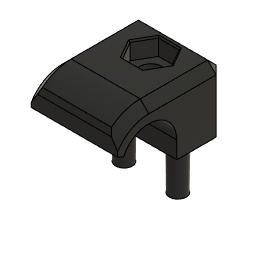
16mm Claw [(P)MPLA000000141] v1 (Autodesk Fusion 360 design; units mm, degrees)
Autodesk Fusion 360 part; units mm, degrees
sketch "Sketch1" plane through (0, 0, 0) normal (1, 0, 0) x (0, 1, 0)
  line L0 (7.7961, -6) -> (22, -6)
  line L1 (8.1, 0) -> (8.1, -8)
  circle A0 centre (0, 0) radius 11.1
  line L2 (0, 11.1) -> (22, 11.1)
  line L3 (22, 11.1) -> (22, -8)
  circle A1 centre (0, 0) radius 8.1
  line L4 (0, 0) -> (-8.1139, 8.1139)
  line L5 (0, 0) -> (-10.06, 4.6911)
  circle A2 centre (0, 0) radius 6.5
  circle A3 centre (0, 0) radius 13.1
  line L6 (-10.06, 4.6911) -> (-10.06, 9.7741)
  line L7 (0, 13.1) -> (22, 13.1)
  line L8 (22, 13.1) -> (22, 11.1)
  line L9 (-9.06, 4.2248) -> (-9.06, 9.7741)
  dimension "d179" = 3
  dimension "d181" = 16.2
  dimension "d182" = 20
  dimension "d6" = 5
  dimension "d33" = 22
  constraint concentric A1 A2
  constraint coincident A0.centre A1.centre
  constraint coincident L2.start A0
  constraint tangent A0 L2
  constraint vertical L3
  constraint coincident L5.end A0
  constraint coincident L0.end L3
  constraint perpendicular L0 L3
  constraint coincident L1.start A1
  constraint tangent L1 A1
  constraint vertical L6
  constraint coincident A3 L7.start
  constraint tangent A3 L7
  constraint perpendicular L3 L7
  constraint perpendicular L2 L8
  constraint parallel L6 L9
  constraint coincident L5 L9.start
  measures "d181" diameter of A1
  measures "d182" angle of L4 L5
  measures "d33" distance of A0.centre L3
extrude "Extrude1" add sketch "Sketch1" along normal mid plane 25 contours L0 L1 A0 A1 L4 | L0 A0 L2 A3 | L0 L2 L3 A3 | A0 A1 L4 L5 L9 | A0 L2 A3 L9 | L2 A3 L7 L8
sketch "Sketch2" plane through (0, 0, -6) normal (0, 0, -1) x (1, 0, 0)
  line L0 (-12.5, -22) -> (12.5, -22)
  line L1 (12.5, -22) -> (12.5, -8.1)
  line L2 (12.5, -8.1) -> (-12.5, -8.1)
  line L3 (-12.5, -8.1) -> (-12.5, -22)
  circle A0 centre (-11.3, 12.8) radius 2.55
  circle A1 centre (-11.3, 12.8) radius 1
  circle A2 centre (4.3, 12.8) radius 2.55
  circle A3 centre (4.3, 12.8) radius 1
  circle A4 centre (0, -13.1) radius 3.2
  circle A5 centre (-7.8, -13.1) radius 2.55
  circle A6 centre (-7.8, -13.1) radius 2.2
  circle A7 centre (7.8, -13.1) radius 2.55
  circle A8 centre (7.8, -13.1) radius 2.2
  dimension "d233" = 2
  dimension "d234" = 2
  dimension "d240" = 15.6
  dimension "d242" = 5.1
  dimension "d243" = 5.1
  dimension "d162" = 6.4
  dimension "d223" = 5.1
  dimension "d224" = 5.1
  dimension "d225" = 4.4
  dimension "d226" = 4.4
  dimension "d227" = 15.6
  dimension "d20" = 7.8
  dimension "d32" = 5
  constraint horizontal A0.centre A2.centre
  constraint concentric A2 A3
  constraint concentric A0 A1
  constraint concentric A7 A8
  constraint concentric A5 A6
  constraint horizontal A7.centre A4.centre
  constraint horizontal A5.centre A4.centre
  constraint vertical origin A4.centre
  measures "d233" diameter of A1
  measures "d234" diameter of A3
  measures "d240" distance of A0.centre A2.centre
  measures "d242" diameter of A2
  measures "d243" diameter of A0
  measures "d162" diameter of A4
  measures "d223" diameter of A7
  measures "d224" diameter of A5
  measures "d225" diameter of A8
  measures "d226" diameter of A6
  measures "d227" distance of A5.centre A7.centre
  measures "d20" distance of A7.centre A4.centre
  measures "d32" distance of L2 A7.centre
extrude "Extrude2" add sketch "Sketch2" along normal blind 12 contours A5 | A6 | A7 | A8
draft "Draft1" angle 0.5 neutral plane through (0, 11.6452, -6) pull (0, 0, -1) 2 faces at (-5.2532, 13.2271, -14) (10.3468, 13.2271, -14)
sketch "Sketch3" plane through (0, 0, -6) normal (0, 0, -1) x (1, 0, 0)
extrude "Extrude3" cut sketch "Sketch2" against normal blind 20 contours A4
sketch "Sketch4" plane through (0, 0, 13.1) normal (0, 0, 1) x (-1, 0, 0)
  circle A0 centre (0, -13.1) radius 3.2
  line L0 (12.5, 0) -> (-12.5, 0)
  line L1 (-12.5, 0) -> (-12.5, -22)
  line L2 (-12.5, -22) -> (12.5, -22)
  line L3 (12.5, -22) -> (12.5, 0)
  line L4 (3.0022, -18.3) -> (6.0044, -13.1)
  line L5 (6.0044, -13.1) -> (3.0022, -7.9)
  line L6 (3.0022, -7.9) -> (-3.0022, -7.9)
  line L7 (-3.0022, -7.9) -> (-6.0044, -13.1)
  line L8 (-6.0044, -13.1) -> (-3.0022, -18.3)
  line L9 (-3.0022, -18.3) -> (3.0022, -18.3)
  point P0 (0, -13.1)
  dimension "d27" = 5.2
  constraint coincident P0 A0.centre
  measures "d27" distance of P0 L9
extrude "Extrude4" cut sketch "Sketch4" against normal blind 5 contours L4 L5 L6 L7 L8 L9
chamfer "Chamfer2" distance 2.5 angle 45 7 edges at (-12.5, 22, 3.55) (12.5, 22, 3.55) (0, 22, 13.1) (12.5, 11, 13.1) (12.5, -4.8816, 12.1565) (-12.5, 11, 13.1) (-12.5, -4.8816, 12.1565)
chamfer "Chamfer1" distance 1 angle 45 7 edges at (0, -9.06, 9.4618) (12.5, 13.8, -6) (0, 8.1, -6) (0, 22, -6) (-12.5, 13.8, -6) (11.25, 20.75, -6) (-11.25, 20.75, -6)
chamfer "Chamfer3" distance 0.4 angle 45 6 edges at (4.5033, 15.7, 13.1) (0, 18.3, 13.1) (-4.5033, 15.7, 13.1) (-4.5033, 10.5, 13.1) (0, 7.9, 13.1) (4.5033, 10.5, 13.1)
equation "d20 = d227 / 2"
